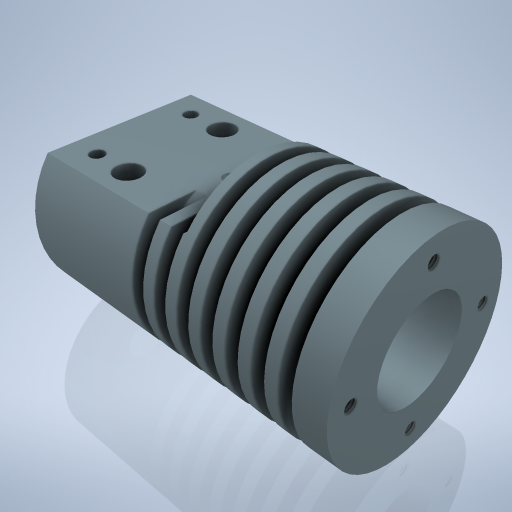
# Autodesk Inventor part: cylinder
Saved by Autodesk Inventor 2024.2 (Build 282272000, 272)
## iProperties
Created: 2024-04-14
Part Number: cylinder
Material: Blei
Document SubType Name: Modeling
Designer: Fabri
Density: 11.34 g/cm^3
Appearance: Blei
Author: Fabri
Autodesk Inventor part; units mm, degrees
note: some values were not read from the file. Chosen so that the rebuilt part matches the saved one: direction of "Bohrung4".
ref_plane "YZ Plane" through (0, 0, 0) normal (1, 0, 0) x (0, 1, 0)
sketch "Skizze3" plane through (0, 0, 0) normal (0, 0, 1) x (1, 0, 0)
  line L0 (0, 0) -> (64, 0)
  line L1 (0, 0) -> (0, 19.5)
  line L2 (0, 19.5) -> (25.5, 19.5)
  line L3 (25.5, 19.5) -> (25.5, 13.5)
  line L4 (25.5, 13.5) -> (28, 13.5)
  line L5 (28, 13.5) -> (28, 19.5)
  line L6 (28, 19.5) -> (30.5, 19.5)
  line L7 (30.5, 19.5) -> (30.5, 13.5)
  line L8 (30.5, 13.5) -> (33, 13.5)
  line L9 (33, 13.5) -> (33, 19.5)
  line L10 (33, 19.5) -> (35.5, 19.5)
  line L11 (35.5, 19.5) -> (35.5, 13.5)
  line L12 (35.5, 13.5) -> (38, 13.5)
  line L13 (38, 13.5) -> (38, 19.5)
  line L14 (38, 19.5) -> (40.5, 19.5)
  line L15 (40.5, 19.5) -> (40.5, 13.5)
  line L16 (40.5, 13.5) -> (43, 13.5)
  line L17 (43, 13.5) -> (43, 19.5)
  line L18 (43, 19.5) -> (45.5, 19.5)
  line L19 (45.5, 19.5) -> (45.5, 13.5)
  line L20 (45.5, 13.5) -> (48, 13.5)
  line L21 (48, 13.5) -> (48, 19.5)
  line L22 (48, 19.5) -> (50.5, 19.5)
  line L23 (50.5, 19.5) -> (50.5, 13.5)
  line L24 (50.5, 13.5) -> (53, 13.5)
  line L25 (53, 13.5) -> (53, 19.5)
  line L26 (53, 19.5) -> (55.5, 19.5)
  line L27 (55.5, 19.5) -> (55.5, 13.5)
  line L28 (55.5, 13.5) -> (58, 13.5)
  line L29 (58, 13.5) -> (58, 19.5)
  line L30 (58, 19.5) -> (64, 19.5)
  line L31 (64, 19.5) -> (64, 0)
  dimension "d8" = 64
  dimension "d9" = 64
  dimension "d10" = 32.5
  dimension "d11" = 6
  dimension "d12" = 2.5
  dimension "d13" = 2.5
  dimension "d14" = 2.5
  dimension "d15" = 2.5
  dimension "d16" = 2.5
  dimension "d17" = 2.5
  dimension "d18" = 2.5
  dimension "d19" = 2.5
  dimension "d20" = 2.5
  dimension "d22" = 2.5
  dimension "d23" = 2.5
  dimension "d24" = 27
  dimension "d25" = 39
  constraints: 64 end point, 26 point on line, 17 perpendicular, 3 horizontal alignment, 1 collinear, 1 horizontal, 1 vertical
  measures "d8" distance of L0.start L0.end
  measures "d9" distance between parallel lines of L31 L1
  measures "d10" distance between parallel lines of L29 L3
  measures "d11" distance between parallel lines of L31 L29
  measures "d12" distance between parallel lines of L5 L3
  measures "d13" distance between parallel lines of L7 L5
  measures "d14" distance between parallel lines of L11 L9
  measures "d15" distance of L11.end L12.end
  measures "d16" distance between parallel lines of L29 L27
  measures "d17" distance between parallel lines of L27 L25
  measures "d18" distance between parallel lines of L25 L23
  measures "d19" distance between parallel lines of L23 L21
  measures "d20" distance between parallel lines of L21 L19
  measures "d22" distance between parallel lines of L19 L17
  measures "d23" distance between parallel lines of L17 L15
  measures "d24" diameter of L4.end L0
  measures "d25" diameter of L30.end L0
revolve "Umdrehung1" add sketch "Skizze3" angle 360 about axis through (0, 0, 0) along (1, 0, 0)
sketch "Skizze4" plane through (0, 0, 0) normal (-1, 0, 0) x (0, 0, 1)
  circle A0 centre (0, 0) radius 19.5 projected
  constraints: 1 coincident
hole "Bohrung1" at (0, 0, 0) direction (1, 0, 0) diameter 8 depth 24.435
sketch "Skizze5" plane through (0, 0, 0) normal (-1, 0, 0) x (0, 0, 1)
  circle A0 centre (0, 0) radius 19.5 projected
  constraints: 1 coincident
hole "Bohrung2" at (0, 0, 0) direction (1, 0, 0) diameter 10 depth 8
sketch "Skizze6" plane through (0, 0, 0) normal (-1, 0, 0) x (0, 0, 1)
  circle A0 centre (0, 0) radius 19.5 projected
  constraints: 1 coincident
hole "Bohrung3" at (0, 0, 0) direction (1, 0, 0) diameter 12 depth 6
ref_plane "Arbeitsebene1" through (0, 0, 0) normal (0, 0, 1) x (1, 0, 0)
sketch "Skizze7" plane through (0, 0, 0) normal (0, 0, 1) x (1, 0, 0)
  line L0 (24.435, 4) -> (24.435, -4) projected
  arc A0 (47.12, 9.5) -> (24.435, 4) centre (46.1397, -35.9894) ccw
  line L1 (64, -19.5) -> (64, 19.5) projected
  line L2 (0, 0) -> (66.8776, 0)
  line L3 (47.12, 9.5) -> (64, 9.5)
  point P0 (64, 10.0584)
  point P1 (24.435, 0)
  point P2 (64, 0)
  dimension "d51" = 45.5
  dimension "d53" = 19
  dimension "d54" = 16.88
  constraints: 4 end point, 2 point on circle, 2 point on line, 1 centre point, 1 horizontal, 1 perpendicular
  measures "d51" radius of A0
  measures "d53" diameter of L3.end L2
  measures "d54" distance of L3.start L3.end
revolve "Umdrehung2" cut sketch "Skizze7" angle 360 about axis through (0, 0, 0) along (1, 0, 0)
sketch "Skizze8" plane through (0, 0, 0) normal (-1, 0, 0) x (0, 0, 1)
  circle A0 centre (0, 0) radius 19.5 projected
  line L0 (12, 15.3704) -> (12, -15.3704)
  dimension "d55" = 12
  constraints: 2 end point, 2 point on circle, 1 vertical
  measures "d55" distance from line of L0 point (0, 0)
extrude "Extrusion1" cut sketch "Skizze8" against normal blind 33.5 contours A0 L0 picked at (14.5, 0)
sketch "Skizze9" plane through (0, -15.3704, 12) normal (0, 0, 1) x (1, 0, 0)
  line L0 (0, 0) -> (0, 30.7409) projected
  line L1 (0, 15.3704) -> (72.1988, 15.3704) construction
  point P0 (14, 25.3704)
  point P1 (14, 5.3704)
  dimension "d65" = 14
  dimension "d66" = 20
  constraints: 2 end point, 1 horizontal, 1 symmetric about line, 1 vertical alignment
  measures "d65" distance from line of point (14, 25.37) L0
  measures "d66" distance of point (14, 5.37) point (14, 25.37)
hole "Bohrung4" at (14, 10, 12) at (14, -10, 12) direction (0, 0, -1) diameter 5.5 end up to surface
sketch "Skizze10" plane through (0, -15.3704, 12) normal (0, 0, 1) x (1, 0, 0)
  line L0 (0, 15.3704) -> (72.7921, 15.3704) construction
  line L1 (0, 0) -> (0, 30.7409) projected
  point P0 (6, 5.3704)
  point P1 (6, 25.3704)
  dimension "d74" = 20
  dimension "d75" = 6
  constraints: 2 end point, 1 horizontal, 1 symmetric about line
  measures "d74" distance of point (6, 5.37) point (6, 25.37)
  measures "d75" distance from line of point (6, 25.37) L1
hole "Bohrung5" at (6, -10, 12) at (6, 10, 12) direction (0, 0, -1) diameter 3 depth 8
sketch "Skizze11" plane through (0, -15.3704, 12) normal (0, 0, 1) x (1, 0, 0)
  line L0 (0, 0) -> (0, 30.7409) projected
  point P0 (0, 15.3704)
  point P1 (26.5, 15.3704)
  point P2 (0, 15.3704)
  dimension "d83" = 26.5
  constraints: 1 horizontal alignment, 1 midpoint
  measures "d83" distance from line of point (26.5, 15.37) L0
hole "Bohrung6" at (26.5, 0, 12) direction (0, 0, -1) diameter 3 depth 19.5
sketch "Skizze12" plane through (64, 0, 0) normal (1, 0, 0) x (0, 0, -1)
  circle A0 centre (0, 0) radius 15 construction
  point P0 (15, 0)
  point P1 (0, 15)
  point P2 (0, -15)
  point P3 (-15, 0)
  dimension "d84" = 30
  constraints: 4 point on circle, 1 centre point, 1 coincident
  measures "d84" diameter of A0
hole "Bohrung7" at (64, 0, -15) at (64, 15, 0) at (64, -15, 0) at (64, 0, 15) direction (-1, 0, 0) diameter 2.459 depth 6 thread size "M3x0.5" class "6H" standard "ISO Metric profile"
ref_plane "Arbeitsebene2" through (0, 0, -19.5) normal (0, 0, 1) x (1, 0, 0)
sketch "Skizze14" plane through (0, 0, -19.5) normal (0, 0, 1) x (1, 0, 0)
  line L0 (0, -19.5) -> (0, 19.5) projected
  point P0 (0, 0)
  point P1 (14, 0)
  point P2 (0, -15.3704)
  point P3 (0, 15.3704)
  dimension "d93" = 14
  constraints: 1 horizontal alignment
  measures "d93" distance from line of L0 point (14, 0)
hole "Bohrung8" at (14, 0, -19.5) direction (0, 0, 1) diameter 5.5 depth 17.5 counterbore diameter 10 counterbore depth 14
equation "\"d18\" = d17"
equation "\"d19\" = d17"
equation "\"d20\" = d18"
equation "\"d22\" = d19"
equation "\"d23\" = d20"
